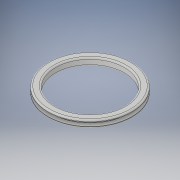
# Autodesk Inventor part: 18mm_id_2mm_height
Saved by Autodesk Inventor 2017 (Build 210142000, 142)
## iProperties
Created: 2016-08-19
Part Number: 18mm_id_2mm_height
Material: Generic
Document SubType Name: Modeling
Designer: jvoigts
Density: 1 g/cm^3
Appearance: Default
Author: jvoigts
Autodesk Inventor part; units mm, degrees
ref_plane "YZ Plane" through (0, 0, 0) normal (1, 0, 0) x (0, 1, 0)
ref_plane "XZ Plane" through (0, 0, 0) normal (0, 1, 0) x (-1, 0, 0)
ref_plane "XY Plane" through (0, 0, 0) normal (0, 0, 1) x (1, 0, 0)
sketch "Sketch1" plane through (0, 0, 0) normal (1, 0, 0) x (0, 1, 0)
  line L0 (-0.9826, 9.0015) -> (1.0174, 9.0015)
  line L1 (1.0174, 9.0015) -> (1.0174, 11.0015)
  line L2 (1.0174, 11.0015) -> (0.4816, 11.0015)
  line L3 (0.4816, 11.0015) -> (0.4816, 9.4702)
  line L4 (0.4816, 9.4702) -> (-0.4886, 9.4702)
  line L5 (-0.4886, 9.4702) -> (-0.4886, 11.0015)
  line L6 (-0.4886, 11.0015) -> (-0.9826, 11.0015)
  line L7 (1.4983, 0) -> (1.4983, 9) construction
  line L8 (-0.9826, 11.0015) -> (-0.9826, 9.0015)
  line L9 (8.3035, 0) -> (4.0958, 0) construction
  point P0 (0, 0)
  dimension "d0" = 9
  dimension "d1" = 2
  dimension "d2" = 2
  constraints: 20 end point, 5 perpendicular, 2 horizontal, 2 point on line, 2 vertical
  measures "d0" distance of L7.start L7.end
  measures "d1" distance of L0.start L0.end
  measures "d2" distance of L0.end L1.end
revolve "Revolution1" add sketch "Sketch1" angle 360 about axis through (0, 8.3035, 0) along (0, -1, 0)
fillet "Fillet2" radius 0.4 6 edges at (0, 1.0174, -9.0015) (0, -0.9826, -9.0015) (0, 1.0174, -11.0015) (0, -0.9826, -11.0015) (0, -0.4886, -9.4702) (0, 0.4816, -9.4702)
body "Solid1"
